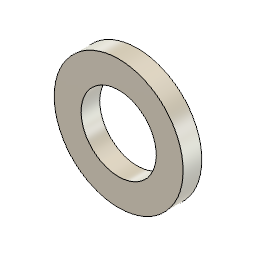
Bike Trainer (Autodesk Fusion 360 archive; units mm, degrees)
design "Washer DIN 433-1 - 6.4 - A Steel 100 HV Plain"
description: Washer DIN 433-1 - 6.4 - A
part number: DIN 433 - 6.4 Steel 100 HV Plain
Autodesk Fusion 360 part; units mm, degrees
sketch "Sketch1" plane through (0, 0, 0) normal (0, 0, 1) x (1, 0, 0)
  circle A0 centre (0, 0) radius 5.5
  circle A1 centre (0, 0) radius 3.2
  dimension "d4" = 11
  dimension "d5" = 6.4
  constraint coincident A0.centre A1.centre
  measures "d4" diameter of A0
  measures "d5" diameter of A1
extrude "Extrude1" add sketch "Sketch1" along normal blind 1.6
equation "adsk_woutdia = 11.00 mm"
equation "adsk_windia = 6.40 mm"
equation "adsk_wthick = 1.60 mm"
equation "d4 = adsk_woutdia"
equation "d5 = adsk_windia"
equation "d6 = adsk_wthick"
equation "d30 = adsk_wthick"

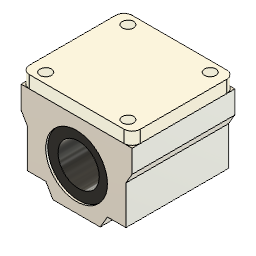
design "SC20 SCS20UU Linear Rail Bearing v2"
Autodesk Fusion 360 part; units mm, degrees
sketch "Sketch1" plane through (0, 0, 0) normal (0, 0, 1) x (1, 0, 0)
  line L0 (0, 0) -> (-27, 0)
  circle A0 centre (0, 21) radius 10
  line L1 (-27, 0) -> (-27, 11)
  line L2 (-24, 35) -> (-15, 35)
  line L3 (-24, 16.1158) -> (-24, 35)
  circle A1 centre (0, 21) radius 15
  line L4 (0, 0) -> (0, 41) construction
  line L5 (0, 0) -> (27, 0)
  line L6 (27, 0) -> (27, 11)
  line L7 (24, 16.1158) -> (24, 35)
  line L8 (24, 35) -> (15, 35)
  line L9 (-15, 35) -> (-15, 0) construction
  line L10 (-27, 11) -> (-24, 16.1158)
  line L11 (-15, 35) -> (-11.4815, 41)
  line L12 (24, 16.1158) -> (27, 11)
  line L13 (11.4815, 41) -> (15, 35)
  line L14 (0, 41) -> (-11.4815, 41)
  line L15 (0, 41) -> (11.4815, 41)
  point P0 (0, 21)
  point P1 (0, 21)
  point P2 (0, 21)
  dimension "d18" = 21
  dimension "d21" = 11
  dimension "d22" = 35
  dimension "d23" = 24
  dimension "d26" = 20
  dimension "d27" = 30
  dimension "d28" = 27
  dimension "d29" = 41
  constraint coincident P2 P0
  constraint horizontal L0
  constraint perpendicular L0 L1
  constraint parallel L1 L3
  constraint perpendicular L1 L2
  constraint coincident P2 P1
  constraint coincident L0.start L4.start
  constraint symmetric L11.end L4 L13.start
  constraint symmetric L2.start L4 L7.end
  constraint symmetric L3.start L4 L7.start
  constraint symmetric L0.start L4 L5.start
  constraint symmetric L0.end L4 L5.end
  constraint symmetric L1.end L4 L6.end
  constraint symmetric L2.end L4 L8.end
  constraint vertical L4
  constraint coincident L0 L9.end
  constraint vertical L9
  constraint coincident P2 L4
  constraint parallel L10 L11
  constraint perpendicular L4 L14
  constraint symmetric L14.start L4 L15.start
  constraint tangent A1 L9
  measures "d18" distance of P2 L0
  measures "d21" distance of L1.end L0
  measures "d22" distance of L0 L2
  measures "d23" distance of L3 L4
  measures "d26" diameter of A0
  measures "d27" diameter of A1
  measures "d28" distance of L1 L4
  measures "d29" distance of L0 L14
extrude "Extrude1" add sketch "Sketch1" along normal mid plane 50 contours L0 L1 L2 L3 L5 L6 L7 L8 L10 L11 L12 L13 L14 L15 makes body 1
extrude "Extrude2" add sketch "Sketch1" along normal mid plane 48 separate body contours A1 makes body 2
sketch "Sketch2" plane through (0, 0, 0) normal (0, -1, 0) x (1, 0, 0)
  line L0 (27, -25) -> (27, 25)
  line L1 (27, 25) -> (-27, 25)
  line L2 (-27, 25) -> (-27, -25)
  line L3 (-27, -25) -> (27, -25)
  line L4 (0, 25) -> (0, -25) construction
  line L5 (-27, 0) -> (27, 0) construction
  point P0 (-20, 20)
  point P1 (20, 20)
  point P2 (-20, -20)
  point P3 (20, -20)
  dimension "d34" = 40
  dimension "d35" = 40
  constraint midpoint L1 L4.start
  constraint midpoint L3 L4.end
  constraint midpoint L2 L5.start
  constraint midpoint L0 L5.end
  constraint symmetric L4 P0 P1
  constraint symmetric L5 P0 P2
  constraint symmetric L5 P1 P3
  measures "d34" distance of P0 P1
  measures "d35" distance of P0 P2
hole "Hole1" at (-20, 0, 20) at (20, 0, 20) at (20, 0, -20) at (-20, 0, -20) direction (0, 1, 0) diameter 5.035 end up to surface (35 mm away) bodies 1
thread "Thread1" "ISO Metric profile 6.0 M6x1 6H" thread offset 0 thread depth 10
move_body "Move1" bodies 2 1 to x (-1, 0, 0) y (0, -1, 0) z (0, 0, 1) at (-51, 27.1158, 0)
sketch "Sketch3" plane through (0, 27.1158, 0) normal (0, 1, 0) x (-1, 0, 0)
  circle A0 centre (71, -20) radius 2.5175
  circle A1 centre (31, 20) radius 2.5175
  circle A2 centre (71, 20) radius 2.5175
  circle A3 centre (31, -20) radius 2.5175
  line L0 (78, -25) -> (78, 25)
  line L1 (78, 25) -> (24, 25)
  line L2 (24, 25) -> (24, -25)
  line L3 (24, -25) -> (78, -25)
  line L4 (74, -25) -> (28, -25)
  line L5 (24, -21) -> (24, 21)
  line L6 (28, 25) -> (74, 25)
  line L7 (78, 21) -> (78, -21)
  circle A4 centre (71, -20) radius 2.75
  circle A5 centre (31, -20) radius 2.75
  circle A6 centre (71, 20) radius 2.75
  circle A7 centre (31, 20) radius 2.75
  arc A8 (74, -25) -> (78, -21) centre (74, -21) ccw
  arc A9 (24, -21) -> (28, -25) centre (28, -21) ccw
  arc A10 (28, 25) -> (24, 21) centre (28, 21) ccw
  arc A11 (78, 21) -> (74, 25) centre (74, 21) ccw
  dimension "d47" = 5.5
  dimension "d48" = 5.5
  dimension "d49" = 5.5
  dimension "d50" = 5.5
  dimension "d51" = 4
  constraint horizontal L4
  constraint vertical L5
  constraint horizontal L6
  constraint vertical L7
  constraint concentric A0 A4
  constraint concentric A3 A5
  constraint concentric A2 A6
  constraint concentric A1 A7
  constraint tangent L4 A8
  constraint tangent L7 A8
  constraint tangent L4 A9
  constraint tangent L5 A9
  constraint equal A8 A9
  constraint tangent L5 A10
  constraint tangent L6 A10
  constraint equal A8 A10
  constraint tangent L6 A11
  constraint tangent L7 A11
  constraint equal A8 A11
  measures "d47" diameter of A4
  measures "d48" diameter of A5
  measures "d49" diameter of A6
  measures "d50" diameter of A7
  measures "d51" radius of A8
extrude "Extrude3" add sketch "Sketch3" along normal blind 6 separate body contours L0 L1 L2 L3 L4 L5 L6 L7 A8 A9 A10 A11 makes body 3
equation "h = 21 mm"
equation "DE = 27 mm"
equation "W1 = DE * 2"
equation "H1F = 41 mm"
equation "G = 35 mm"
equation "A1T = 11 mm"
equation "B = 40 mm"
equation "d18 = h"
equation "d21 = A1T"
equation "d22 = G"
equation "d23 = DE - 3 mm"
equation "Dia = 20 mm"
equation "Dia2 = Dia + 10 mm"
equation "d26 = Dia"
equation "d27 = Dia2"
equation "d28 = DE"
equation "d29 = H1F"
equation "d30 = L"
equation "d32 = L2"
equation "d34 = B"
equation "d35 = C1"
equation "C1 = 40 mm"
equation "L = 50 mm"
equation "L2 = L - 2 mm"
equation "S2 = 6 mm"
named bodies: "Spacer"
